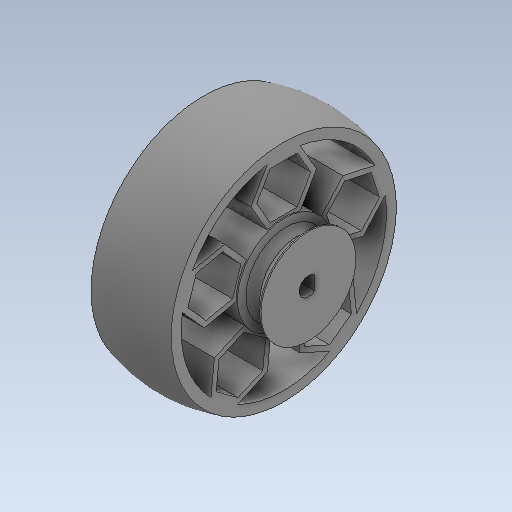
# Autodesk Inventor part: PulleyedWheelV1
Saved by Autodesk Inventor 2020 (Build 240168000, 168)
## iProperties
Created: 2023-12-21
Part Number: PulleyedWheelV1
Material: H TPU
Document SubType Name: Modeling
Designer: smz3rm
Density: 0.941117 g/cm^3
Appearance: Generic(1)
Mass: 7.7724 g
Surface Area: 68.3098 cm^2
Volume: 8.2587 cm^3
d0: 3.000 mm
d1: 1.000 mm
d3: 36.500 mm
d4: 3.000 mm
d6: 15.400 mm
d7: 4.000 mm
d8: 0.00 deg
d9: 36.500 mm
d10: 1.600 mm
d11: 0.800 mm
d16: 13.000 mm
d17: 0.00 deg
d20: 2.000 mm
d24: 1.000 mm
d26: 45.00 deg
Roundedness: 1.000 mm
BaseThickness: 3.000 mm
TopThickness: 1.778 mm
SideThickness: 4.000 mm
BodyWidth: 130.000 mm
BodyLength: 150.000 mm
BodyHeight: 35.000 mm
DriveMotorHeight: 17.500 mm
WheelDia: 38.500 mm
WheelWidth: 13.000 mm
WheelGrooveWidth: 4.000 mm
WheelGrooveDia: 15.400 mm
WheelSlotWidth: 20.000 mm
WheelPulleyDia: 2.000 mm
WheeGuardlSlotWidth: 20.000 mm
Author: smz3rm
Autodesk Inventor part; units mm, degrees
ref_plane "YZ Plane" through (0, 0, 0) normal (1, 0, 0) x (0, 1, 0)
ref_plane "XZ Plane" through (0, 0, 0) normal (0, 1, 0) x (-1, 0, 0)
ref_plane "XY Plane" through (0, 0, 0) normal (0, 0, 1) x (1, 0, 0)
sketch "Sketch1" plane through (0, 0, 0) normal (1, 0, 0) x (0, 1, 0)
  circle A0 centre (0, 0) radius 1.5
  line L0 (-24.15, 0) -> (24.15, 0) projected
  line L1 (1.118, -1) -> (-1.118, -1)
  circle A1 centre (0, 0) radius 7.7
  circle A2 centre (0, 0) radius 18.25
  circle A3 centre (0, 0) radius 15.25
  dimension "d0" = 3
  dimension "d1" = 1
  dimension "d3" = 36.5
  dimension "d4" = 3
  dimension "d6" = 15.4
  constraints: 4 centre point, 4 coincident, 2 end point, 2 point on circle, 1 horizontal
  measures "d0" diameter of A0
  measures "d1" distance between parallel lines of L0 L1
  measures "d3" diameter of A2
  measures "d4" radial gap between concentric circles of A2 A3
  measures "d6" diameter of A1
extrude "Extrusion1" add sketch "Sketch1" along normal blind 4 contours L1 A0 | A0 L0 A1 | L0 A1 A0
sketch "Sketch3" plane through (0, 0, 0) normal (0, 0, 1) x (1, 0, 0)
  line L0 (0, 7.7) -> (4, 7.7) projected
  line L1 (-0.8, 0) -> (4.8, 0) projected
  circle A0 centre (1.3858, 6.7) radius 1
  line L2 (0.4001, 6.5312) -> (0.2, 7.7)
  line L3 (0, 7.7) -> (4, 7.7) projected
  line L4 (0, 10) -> (4, 10) projected
  line L5 (0, 7.7) -> (4, 7.7) projected
  line L6 (3.8, 7.7) -> (2.0929, 5.9929)
  line L7 (3.8, 7.7) -> (3.8, 7.7)
  line L8 (3.8, 7.7) -> (4, 7.7)
  line L9 (4, -7.7) -> (4, 7.7) projected
  line L10 (4, 7.7) -> (4, 7.7)
  line L11 (0, -7.7) -> (0, 7.7) projected
  line L12 (0.2, 7.7) -> (0, 7.7)
  point P0 (0, 0)
  point P1 (1.3858, 7.7)
  point P2 (3.8, 7.7)
  dimension "d20" = 2
  dimension "d26" = 45
  dimension "d28" = 0.2
  constraints: 12 end point, 3 perpendicular, 3 tangent, 2 collinear, 2 point on circle, 2 point on line, 1 centre point, 1 vertical, 3 other
  measures "d20" diameter of A0
  measures "d26" angle of L0 L6
  measures "d28" distance of L0.end L6.start
revolve "Revolution1" cut sketch "Sketch3" angle 360 about axis through (-10, 0, 0) along (-1, 0, 0) contours L0 A0 L2 | L0 L6 A0 | A0
sketch "Sketch2" plane through (0, 0, 0) normal (-1, 0, 0) x (0, 0, 1)
  circle A0 centre (0, 0) radius 18.25
  circle A1 centre (0, 0) radius 16.65
  circle A2 centre (0, 0) radius 7.7 projected
  line L0 (-1, 1.118) -> (-1, -1.118) projected
  arc A3 (-1, -1.118) -> (-1, 1.118) centre (0, 0) ccw projected
  line L1 (2.6587, 16.4364) -> (5.3173, 11.8314)
  line L2 (5.3173, 11.8314) -> (2.6587, 7.2264)
  line L3 (2.6587, 7.2264) -> (-2.6587, 7.2264)
  line L4 (-2.6587, 7.2264) -> (-5.3173, 11.8314)
  line L5 (-5.3173, 11.8314) -> (-2.6587, 16.4364)
  line L6 (-2.6587, 16.4364) -> (2.6587, 16.4364)
  line L7 (0, -24.15) -> (0, 24.15) projected
  line L8 (-2.1968, 15.6364) -> (-4.3936, 11.8314)
  line L9 (-4.3936, 11.8314) -> (-2.1968, 8.0264)
  line L10 (-2.1968, 8.0264) -> (2.1968, 8.0264)
  line L11 (2.1968, 8.0264) -> (4.3936, 11.8314)
  line L12 (4.3936, 11.8314) -> (2.1968, 15.6364)
  line L13 (2.1968, 15.6364) -> (-2.1968, 15.6364)
  line L14 (-14.8103, 7.6077) -> (-9.6092, 8.7132)
  line L15 (-16.4535, 2.5506) -> (-14.8103, 7.6077)
  line L16 (-12.8955, -1.401) -> (-16.4535, 2.5506)
  line L17 (-7.6943, -0.2955) -> (-12.8955, -1.401)
  line L18 (-12.61, -0.5224) -> (-8.3124, 0.391)
  line L19 (-8.3124, 0.391) -> (-6.9548, 4.5696)
  line L20 (-6.9548, 4.5696) -> (-9.8946, 7.8347)
  line L21 (-9.6092, 8.7132) -> (-6.0512, 4.7616)
  line L22 (-6.0512, 4.7616) -> (-7.6943, -0.2955)
  line L23 (-9.8946, 7.8347) -> (-14.1922, 6.9212)
  line L24 (-14.1922, 6.9212) -> (-15.5499, 2.7426)
  line L25 (-15.5499, 2.7426) -> (-12.61, -0.5224)
  line L26 (-11.812, -11.7346) -> (-11.2561, -6.4463)
  line L27 (-7.5101, -14.86) -> (-11.812, -11.7346)
  line L28 (-2.6525, -12.6973) -> (-7.5101, -14.86)
  line L29 (-2.0967, -7.409) -> (-2.6525, -12.6973)
  line L30 (-3.3998, -12.1543) -> (-2.9406, -7.7848)
  line L31 (-2.9406, -7.7848) -> (-6.4951, -5.2023)
  line L32 (-6.4951, -5.2023) -> (-10.5088, -6.9893)
  line L33 (-11.2561, -6.4463) -> (-6.3985, -4.2836)
  line L34 (-6.3985, -4.2836) -> (-2.0967, -7.409)
  line L35 (-10.5088, -6.9893) -> (-10.9681, -11.3588)
  line L36 (-10.9681, -11.3588) -> (-7.4136, -13.9413)
  line L37 (-7.4136, -13.9413) -> (-3.3998, -12.1543)
  line L38 (7.5101, -14.86) -> (2.6525, -12.6973)
  line L39 (11.812, -11.7346) -> (7.5101, -14.86)
  line L40 (11.2561, -6.4463) -> (11.812, -11.7346)
  line L41 (6.3985, -4.2836) -> (11.2561, -6.4463)
  line L42 (10.5088, -6.9893) -> (6.4951, -5.2023)
  line L43 (6.4951, -5.2023) -> (2.9406, -7.7848)
  line L44 (2.9406, -7.7848) -> (3.3998, -12.1543)
  line L45 (2.6525, -12.6973) -> (2.0967, -7.409)
  line L46 (2.0967, -7.409) -> (6.3985, -4.2836)
  line L47 (3.3998, -12.1543) -> (7.4136, -13.9413)
  line L48 (7.4136, -13.9413) -> (10.9681, -11.3588)
  line L49 (10.9681, -11.3588) -> (10.5088, -6.9893)
  line L50 (16.4535, 2.5506) -> (12.8955, -1.401)
  line L51 (14.8103, 7.6077) -> (16.4535, 2.5506)
  line L52 (9.6092, 8.7132) -> (14.8103, 7.6077)
  line L53 (6.0512, 4.7616) -> (9.6092, 8.7132)
  line L54 (9.8946, 7.8347) -> (6.9548, 4.5696)
  line L55 (6.9548, 4.5696) -> (8.3124, 0.391)
  line L56 (8.3124, 0.391) -> (12.61, -0.5224)
  line L57 (12.8955, -1.401) -> (7.6943, -0.2955)
  line L58 (7.6943, -0.2955) -> (6.0512, 4.7616)
  line L59 (12.61, -0.5224) -> (15.5499, 2.7426)
  line L60 (15.5499, 2.7426) -> (14.1922, 6.9212)
  line L61 (14.1922, 6.9212) -> (9.8946, 7.8347)
  point P0 (0, 11.8314)
  point P1 (2.6587, 7.2264)
  point P2 (-14.8103, 7.6077)
  point P3 (-6.0512, 4.7616)
  point P4 (-16.4535, 2.5506)
  point P5 (-7.6943, -0.2955)
  point P6 (-6.3985, -4.2836)
  point P7 (-11.812, -11.7346)
  point P8 (-7.5101, -14.86)
  point P9 (-2.0967, -7.409)
  point P10 (2.0967, -7.409)
  point P11 (7.5101, -14.86)
  point P12 (11.812, -11.7346)
  point P13 (6.3985, -4.2836)
  point P14 (7.6943, -0.2955)
  point P15 (16.4535, 2.5506)
  point P16 (14.8103, 7.6077)
  point P17 (6.0512, 4.7616)
  dimension "d9" = 36.5
  dimension "d10" = 1.6
  dimension "d11" = 0.8
  dimension "d31" = 360
  constraints: 120 end point, 2 centre point, 2 coincident, 2 point on circle, 1 point on line, 141 other
  measures "d9" diameter of A0
  measures "d10" radial gap between concentric circles of A0 A1
  measures "d11" distance between parallel lines of L5 L8
extrude "Extrusion2" add sketch "Sketch2" along normal blind 13 contours A0 L7 A1 | L7 A1 A0 | L7 L6 A1 | A1 L6 L7 | L1 L2 A2 L7 L10 L11 L12 L13 L6 | L6 L7 L13 L8 L9 L10 A2 L4 L5 | A1 L27 | L27 L26 L33 A2 L29 L28 | L39 A1 | L38 L45 A2 L41 L40 L39 | L7 A3 L3 A2 L58 L46 | A2 L34 L22 L3 L7 A3 L0 | A1 L51 | L51 L50 L57 A2 L53 L52 | L15 A1 | L14 L21 A2 L17 L16 L15 | A2 L34 | L46 A2 | L7 A3 | A3 L0 L7 | L3 L7 A2 | A2 L7 L3 | A2 L58 | L22 A2
sketch "Sketch4" plane through (0, 0, 0) normal (0, 0, 1) x (1, 0, 0)
  line L0 (0, 18.25) -> (-13, 18.25) projected
  line L1 (-13, 18.25) -> (-13, -18.25) projected
  arc A0 (0, 18.25) -> (-13, 18.25) centre (-6.5, -2.375) ccw
  line L2 (-15.6, 0) -> (2.6, 0) projected
  point P0 (0, 0)
  point P1 (-6.5, 19.25)
  dimension "d24" = 1
  constraints: 3 point on circle, 1 centre point
  measures "d24" distance from line of L0 point (-6.5, 19.25)
revolve "Revolution2" add sketch "Sketch4" angle 360 about axis through (-10, 0, 0) along (1, 0, 0)
equation "\"d6\" = WheelGrooveDia"
equation "\"d7\" = WheelGrooveWidth"
equation "\"d20\" = WheelPulleyDia"
equation "\"d9\" = WheelDia - 2 * Roundedness"
equation "\"d16\" = WheelWidth"
equation "\"d24\" = Roundedness"
equation "\"Roundedness\" = 1"
equation "\"WheelGrooveDia\" = 15.4"
equation "\"WheelGrooveWidth\" = 4"
equation "\"WheelPulleyDia\" = 2"
equation "\"WheelDia\" = 38.5"
equation "\"WheelWidth\" = 13"
body "Solid1"
